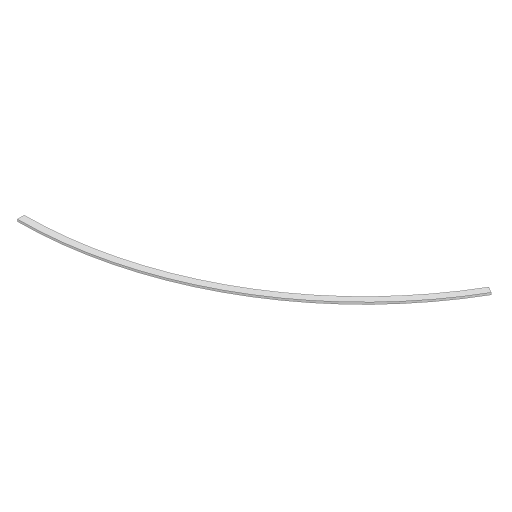
# Autodesk Inventor part: D100_CM_CIRCULO
Saved by Autodesk Inventor 2024.2 (Build 282272000, 272)
## iProperties
Created: 2024-10-01
Part Number: D100_CM_CIRCULO
Material: Generic
Document SubType Name: Modeling
Designer: jrcer
Density: 1 g/cm^3
Appearance: Default
Author: jrcer
Autodesk Inventor part; units mm, degrees
ref_plane "YZ Plane" through (0, 0, 0) normal (1, 0, 0) x (0, 1, 0)
ref_plane "XZ Plane" through (0, 0, 0) normal (0, 1, 0) x (-1, 0, 0)
ref_plane "XY Plane" through (0, 0, 0) normal (0, 0, 1) x (1, 0, 0)
sketch "Sketch1" plane through (0, 0, 0) normal (0, 1, 0) x (-1, 0, 0)
  circle A0 centre (0, 0) radius 500
  circle A1 centre (0, 0) radius 510
  line L0 (510, 0) -> (500, 0)
  line L1 (-510, 0) -> (-500, 0)
  line L2 (0, 0) -> (-433.0127, 250) construction
  line L3 (0, 500) -> (0, 0) construction
  line L4 (0, 510) -> (0, 500)
  line L5 (-433.0127, 250) -> (-441.673, 255)
  point P0 (505, 0)
  point P1 (-505, 0)
  dimension "d0" = 1000
  dimension "d1" = 1020
  dimension "d4" = 60
  constraints: 12 end point, 8 point on circle, 2 centre point, 2 coincident, 2 horizontal, 2 horizontal alignment, 2 midpoint, 2 vertical, 1 collinear
  measures "d0" diameter of A0
  measures "d1" diameter of A1
  measures "d4" angle of L2 L3
extrude "Extrusion1" add sketch "Sketch1" along normal blind 3 contours A0 L5 A1 L4
body "Solid1"
